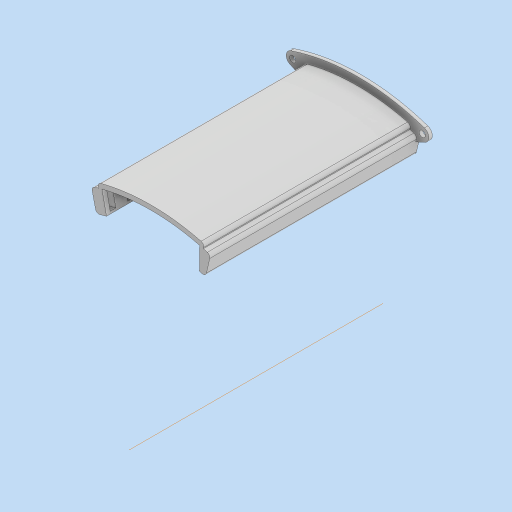
# Autodesk Inventor part: Shim_Tray
Saved by Autodesk Inventor 2024.2 (Build 282272000, 272)
## iProperties
Created: 2025-04-23
Part Number: Shim_Tray
Material: Generic
Document SubType Name: Modeling
Designer: 23661194
Density: 1 g/cm^3
Appearance: Default
Author: 23661194
Autodesk Inventor part; units mm, degrees
ref_plane "YZ Plane" through (0, 0, 0) normal (1, 0, 0) x (0, 1, 0)
ref_plane "XZ Plane" through (0, 0, 0) normal (0, 1, 0) x (-1, 0, 0)
sketch "Shim Tray Slot" plane through (0, 0, 0) normal (0, 0, 1) x (1, 0, 0)
  arc A0 (-28.6337, 111.3782) -> (-30.092, 109.0254) centre (-28.1357, 109.4412) ccw
  arc A1 (-31.6821, 97.1202) -> (-29.1504, 95.657) centre (-29.7334, 97.5701) ccw
  arc A2 (29.1504, 95.657) -> (31.6821, 97.1202) centre (29.7309, 97.5743) ccw
  arc A3 (33.5758, 105.3229) -> (32.2001, 107.689) centre (31.6271, 105.7728) ccw
  arc A4 (30.092, 109.0254) -> (28.6337, 111.3782) centre (28.1357, 109.4412) ccw
  line L0 (30.092, 109.0254) -> (29.9458, 108.3375)
  line L1 (33.5758, 105.3229) -> (31.6821, 97.1202)
  line L2 (-33.5758, 105.3229) -> (-31.6821, 97.1202)
  line L3 (-30.092, 109.0254) -> (-29.9458, 108.3375)
  arc A5 (-32.2001, 107.689) -> (-33.5758, 105.3229) centre (-31.6271, 105.7728) ccw
  arc A6 (29.1504, 95.657) -> (-29.1504, 95.657) centre (0, 0) ccw
  arc A7 (28.6337, 111.3782) -> (-28.6337, 111.3782) centre (0, 0) ccw
  arc A8 (-29.9458, 108.3375) -> (-32.2001, 107.689) centre (0, 0) ccw
  arc A9 (32.2001, 107.689) -> (29.9458, 108.3375) centre (0, 0) ccw
  line L4 (0, 0) -> (0, 107.5)
sketch "Sketch1" plane through (0, 0, 0) normal (0, 0, 1) x (1, 0, 0)
  circle A0 centre (0, 0) radius 100
  circle A1 centre (0, 0) radius 115
  line L0 (0, 161) -> (0, -161) projected
  line L1 (-34.5812, 109.6774) -> (-31.1949, 95.0099)
  line L2 (-161, 0) -> (161, 0) projected
  line L3 (34.5812, 109.6774) -> (31.1949, 95.0099)
  circle A2 centre (0, 0) radius 112.4
  line L4 (-25.4301, 96.7125) -> (-28.0109, 108.8538)
  line L5 (-29.9458, 108.3375) -> (-30.4873, 110.8852)
  arc A3 (-29.9458, 108.3375) -> (-33.9944, 107.1361) centre (0, 0) ccw
  arc A4 (-25.4301, 96.7125) -> (-31.1949, 95.0099) centre (0, 0) ccw
  line L6 (25.4301, 96.7125) -> (28.0109, 108.8538)
  line L7 (29.9458, 108.3375) -> (30.4873, 110.8852)
  arc A5 (31.1949, 95.0099) -> (25.4301, 96.7125) centre (0, 0) ccw
  arc A6 (33.9944, 107.1361) -> (29.9458, 108.3375) centre (0, 0) ccw
  arc A7 (28.0109, 108.8538) -> (-28.0109, 108.8538) centre (0, 0) ccw
  arc A8 (30.4873, 110.8852) -> (-30.4873, 110.8852) centre (0, 0) ccw
  circle A9 centre (0, 0) radius 101.2
  circle A10 centre (0, 0) radius 110.8
  line L8 (28.0109, 108.8538) -> (27.6779, 107.2873)
  line L9 (27.6779, 107.2873) -> (27.7719, 97.3148)
  line L10 (27.7719, 97.3148) -> (27.5218, 96.1382)
  circle A11 centre (0, 0) radius 107.5
  point P0 (0, 107.5)
  dimension "d41" = 202.4
  dimension "d42" = 221.6
  dimension "d53" = 215
  dimension "d0" = 200
  dimension "d1" = 230
  dimension "d4" = 69.1623
  dimension "d5" = 34.5812
  dimension "d6" = 34.5812
  dimension "d7" = 77
  dimension "d8" = 77
  dimension "d9" = 224.8
  dimension "d10" = 6
  dimension "d11" = 78
  dimension "d13" = 2
  dimension "d14" = 6
  dimension "d15" = 78
  dimension "d17" = 2
  dimension "d43" = 0.54
  dimension "d44" = -12
  constraints: 25 point on circle, 18 coincident, 18 end point, 9 centre point, 4 point on line, 1 midpoint, 1 vertical alignment, 8 other
  measures "d0" diameter of A0
  measures "d1" diameter of A1
  measures "d4" distance of L3.start L1.start
  measures "d5" distance from line of L0 L1.start
  measures "d6" distance from line of L0 L3.start
  measures "d7" angle of L2 L1
  measures "d8" angle of L2 L3
  measures "d9" diameter of A2
  measures "d10" distance from line of L4.start L1
  measures "d11" angle of L2 L4
  measures "d13" distance between parallel lines of L4 L5
  measures "d14" distance from line of L6.start L3
  measures "d15" angle of L2 L6
  measures "d17" distance between parallel lines of L6 L7
  measures "d43" angle of L0 L9
  measures "d44" angle of L0 L10
extrude "Extrusion1" add sketch "Sketch1" along normal blind 118 contours A0 L10 A9 L3 | A9 L9 A11 L3 | A11 L9 A10 L3 | L1 A9 L4 A0 | A10 L6 A2 L3 | L1 A11 L4 A9 | L1 A10 L4 A11 | A2 L0 A1 L7 | L1 A2 L4 A10 | A2 L5 A1 L0
fillet "Fillet1" radius 2 6 edges at (-33.9944, 107.1361, 59) (-31.1949, 95.0099, 59) (-30.4873, 110.8852, 59) (30.4873, 110.8852, 59) (33.9944, 107.1361, 59) (31.1949, 95.0099, 59)
ref_plane "Work Plane2" through (0, 0, 5.6) normal (0, 0, 1) x (1, 0, 0)
sketch "Sketch3" plane through (0, 0, 5.6) normal (0, 0, 1) x (1, 0, 0)
  circle A0 centre (0, 0) radius 101.2
  circle A1 centre (0, 0) radius 110.8
  line L0 (-25.4301, 96.7125) -> (-28.0109, 108.8538) projected
  line L1 (-25.6799, 97.8876) -> (-27.6779, 107.2873)
  line L2 (-33.5758, 105.3229) -> (-31.6821, 97.1202) projected
  line L3 (-29.7447, 96.73) -> (-31.9092, 106.1058)
  line L4 (31.6821, 97.1202) -> (33.5758, 105.3229) projected
  line L5 (29.7447, 96.73) -> (31.9092, 106.1058)
  line L6 (27.6779, 107.2873) -> (25.6799, 97.8876)
  line L7 (0, 160.16) -> (0, -155.96) projected
  arc A2 (31.9092, 106.1058) -> (27.6779, 107.2873) centre (0, 0) ccw
  arc A3 (29.7447, 96.73) -> (25.6799, 97.8876) centre (0, 0) ccw
  dimension "d30" = 202.4
  dimension "d31" = 221.6
  dimension "d32" = 1.8
  dimension "d33" = 1.8
  dimension "d45" = 1.8
  dimension "d46" = 1.8
  dimension "d47" = 12
  constraints: 12 point on circle, 8 end point, 4 centre point, 4 coincident, 2 point on line
  measures "d30" diameter of A0
  measures "d31" diameter of A1
  measures "d32" distance from line of L2 L3.start
  measures "d33" distance from line of L2 L3.end
  measures "d45" distance from line of L4 L5.end
  measures "d46" distance from line of L4 L5.start
  measures "d47" angle of L7 L6
extrude "Extrusion3" cut sketch "Sketch3" against normal blind 3.2 contours A0 L6 A1 L5 | L3 A1 L0 A0
fillet "Fillet2" radius 1 2 edges at (-31.9092, 106.1058, 4) (31.9092, 106.1058, 4)
pattern_linear "Rectangular Pattern1" count 12 spacing 10 along (0, 0, 1) of "Extrusion3", "Fillet2"
sketch "Sketch5" plane through (0, 0, 118) normal (0, 0, 1) x (1, 0, 0)
  arc A0 (-25.4301, 96.7125) -> (-29.1504, 95.657) centre (0, 0) ccw projected
  arc A1 (-28.6337, 111.3782) -> (-30.092, 109.0254) centre (-28.1357, 109.4412) ccw projected
  arc A2 (-31.6821, 97.1202) -> (-29.1504, 95.657) centre (-29.7334, 97.5701) ccw projected
  arc A3 (33.5758, 105.3229) -> (32.2001, 107.689) centre (31.6271, 105.7728) ccw projected
  arc A4 (30.092, 109.0254) -> (28.6337, 111.3782) centre (28.1357, 109.4412) ccw projected
  line L0 (29.9458, 108.3375) -> (30.092, 109.0254) projected
  line L1 (-33.5758, 105.3229) -> (-31.6821, 97.1202) projected
  line L2 (-30.092, 109.0254) -> (-29.9458, 108.3375) projected
  arc A5 (-32.2001, 107.689) -> (-33.5758, 105.3229) centre (-31.6271, 105.7728) ccw projected
  line L3 (-25.4301, 96.7125) -> (-28.0109, 108.8538) projected
  arc A6 (28.0109, 108.8538) -> (-28.0109, 108.8538) centre (0, 0) ccw
  arc A7 (-29.9458, 108.3375) -> (-32.2001, 107.689) centre (0, 0) ccw projected
  circle A8 centre (0, 0) radius 107.5
  arc A9 (-28.6337, 111.3782) -> (-30.092, 109.0254) centre (-28.1357, 109.4412) ccw
  arc A10 (-31.6821, 97.1202) -> (-29.1504, 95.657) centre (-29.7334, 97.5701) ccw
  arc A11 (29.1504, 95.657) -> (31.6821, 97.1202) centre (29.7309, 97.5743) ccw
  arc A12 (33.5758, 105.3229) -> (32.2001, 107.689) centre (31.6271, 105.7728) ccw
  arc A13 (30.092, 109.0254) -> (28.6337, 111.3782) centre (28.1357, 109.4412) ccw
  line L4 (30.092, 109.0254) -> (29.9458, 108.3375)
  line L5 (33.5758, 105.3229) -> (31.6821, 97.1202)
  line L6 (-33.5758, 105.3229) -> (-31.6821, 97.1202)
  line L7 (-30.092, 109.0254) -> (-29.9458, 108.3375)
  arc A14 (-32.2001, 107.689) -> (-33.5758, 105.3229) centre (-31.6271, 105.7728) ccw
  arc A15 (29.1504, 95.657) -> (-29.1504, 95.657) centre (0, 0) ccw
  arc A16 (28.6337, 111.3782) -> (-28.6337, 111.3782) centre (0, 0) ccw
  arc A17 (-29.9458, 108.3375) -> (-32.2001, 107.689) centre (0, 0) ccw
  arc A18 (32.2001, 107.689) -> (29.9458, 108.3375) centre (0, 0) ccw
  line L8 (0, 0) -> (0, 107.5)
  dimension "d55" = 215
  constraints: 2 centre point, 2 point on circle, 8 other
  measures "d55" diameter of A8
sketch "Sketch6" plane through (0, 0, 0) normal (0, 0, 1) x (1, 0, 0)
  arc A0 (29.1504, 95.657) -> (27.5218, 96.1382) centre (0, 0) ccw projected
  arc A1 (29.1504, 95.657) -> (-29.1504, 95.657) centre (0, 0) ccw
  arc A2 (28.6337, 111.3782) -> (-28.6337, 111.3782) centre (0, 0) ccw projected
  arc A3 (28.6337, 111.3782) -> (-28.6337, 111.3782) centre (0, 0) ccw
  arc A4 (30.092, 109.0254) -> (28.6337, 111.3782) centre (28.1357, 109.4412) ccw projected
  arc A5 (30.092, 109.0254) -> (28.6337, 111.3782) centre (28.1357, 109.4412) ccw
  arc A6 (33.5758, 105.3229) -> (32.2001, 107.689) centre (31.6271, 105.7728) ccw projected
  arc A7 (33.5758, 105.3229) -> (32.2001, 107.689) centre (31.6271, 105.7728) ccw
  arc A8 (29.1504, 95.657) -> (31.6821, 97.1202) centre (29.7334, 97.5701) ccw projected
  arc A9 (29.1504, 95.657) -> (31.6821, 97.1202) centre (29.7334, 97.5701) ccw
  arc A10 (-31.6821, 97.1202) -> (-29.1504, 95.657) centre (-29.7334, 97.5701) ccw projected
  arc A11 (-31.6821, 97.1202) -> (-29.1504, 95.657) centre (-29.7334, 97.5701) ccw
  arc A12 (-28.6337, 111.3782) -> (-30.092, 109.0254) centre (-28.1357, 109.4412) ccw projected
  arc A13 (-28.6337, 111.3782) -> (-30.092, 109.0254) centre (-28.1357, 109.4412) ccw
  arc A14 (-32.2001, 107.689) -> (-33.5758, 105.3229) centre (-31.6271, 105.7728) ccw projected
  arc A15 (-32.2001, 107.689) -> (-33.5758, 105.3229) centre (-31.6271, 105.7728) ccw
  arc A16 (32.2001, 107.689) -> (29.9458, 108.3375) centre (0, 0) ccw projected
  line L0 (32.2001, 107.689) -> (29.9458, 108.3375)
  line L1 (29.9458, 108.3375) -> (30.092, 109.0254)
  line L2 (33.5758, 105.3229) -> (31.6821, 97.1202)
  line L3 (-33.5758, 105.3229) -> (-31.6821, 97.1202) projected
  line L4 (-31.6821, 97.1202) -> (-33.5758, 105.3229)
  line L5 (-30.092, 109.0254) -> (-29.9458, 108.3375) projected
  line L6 (-30.092, 109.0254) -> (-29.9458, 108.3375)
  arc A17 (-29.9458, 108.3375) -> (-32.2001, 107.689) centre (0, 0) ccw projected
  line L7 (-29.9458, 108.3375) -> (-32.2001, 107.689)
  arc A18 (47.2152, 105.6825) -> (0, 115.75) centre (0, 0) ccw
  circle A19 centre (37, 109.6771) radius 1.75
  arc A20 (0, 115.75) -> (-45.3069, 106.5145) centre (0, 0) ccw
  circle A21 centre (-37, 109.6771) radius 1.75
  line L8 (0, 163.6931) -> (0, -152.6989) projected
  circle A22 centre (37, 109.6771) radius 3.75
  circle A23 centre (-37, 109.6771) radius 3.75
  line L9 (0, 0) -> (37, 109.6771)
  line L10 (37, 109.6771) -> (38.1987, 113.2303)
  line L11 (0, 0) -> (-37, 109.6771)
  arc A24 (38.1987, 113.2303) -> (-38.1987, 113.2303) centre (0, 0) ccw
  circle A25 centre (0, 0) radius 109
  line L12 (33.2271, 103.8122) -> (38, 106.0629)
  line L13 (-33.2271, 103.8122) -> (-38, 106.0629)
  point P0 (-33.2271, 103.8122)
  point P1 (27.5218, 96.1382)
  dimension "d56" = 115.75
  dimension "d57" = 3.5
  dimension "d58" = 3.5
  dimension "d59" = 37
  dimension "d60" = 37
  dimension "d61" = 7.5
  dimension "d62" = 7.5
  dimension "d63" = 218
  constraints: 31 point on circle, 22 end point, 16 centre point, 13 coincident, 2 collinear, 2 point on line
  measures "d56" radius of A18
  measures "d57" diameter of A19
  measures "d58" diameter of A21
  measures "d59" distance from line of L8 A19.centre
  measures "d60" distance from line of L8 A21.centre
  measures "d61" diameter of A22
  measures "d62" diameter of A23
  measures "d63" diameter of A25
extrude "Extrusion4" add sketch "Sketch6" against normal blind 2 contours A0 A1 L8 A25 L2 A8 | A1 A10 L3 A25 L8 | A25 L8 A2 A4 L1 L0 A6 L2 | L2 A6 A16 L1 A4 A2 L8 A18 A22 L9 L12 | A25 L3 A14 L7 L5 A12 A2 L8 | L9 A22 L12 | A2 A12 L5 A17 A14 L3 L13 L11 A23 A20 L8 | L0 A16 | L9 A19 A18 A22 | A22 A18 A19 L9 | L8 A24 A22 A18 | A20 A23 A24 L8 | L13 A23 L11 | A22 L10 A19 A18 | A18 A19 L10 A22 | A23 L11 A21 A20 | A20 A21 A23 | A17 L7 | A23 A20 A21 L11
sketch "Sketch7" plane through (0, 0, 0) normal (0, 0, 1) x (1, 0, 0)
  arc A0 (27.5218, 96.1382) -> (-25.4301, 96.7125) centre (0, 0) ccw projected
  line L0 (0, 164.9) -> (0, -152.9) projected
  line L1 (0, 100) -> (-6.0909, 111.9541)
  line L2 (0, 100) -> (6.0909, 111.9541)
  arc A1 (6.0909, 111.9541) -> (-6.0909, 111.9541) centre (0, 0) ccw
  point P0 (0, 100)
  dimension "d67" = 27
  dimension "d69" = 27
  constraints: 4 end point, 3 point on circle, 2 point on line, 1 centre point, 1 coincident
  measures "d67" angle of L0 L1
  measures "d69" angle of L0 L2
extrude "Extrusion5" cut sketch "Sketch7" against normal blind 2
thicken "Thicken1" operation cut thickness 0.5 both sides no extend neighbours no toward (0.8910065, -0.4539905, 0) faces at (2.0303, 103.9847, -0.6667) (-4.0606, 107.9694, -0.6667)
fillet "Fillet3" radius 1 6 edges at (0.5604, 99.9984, -1) (-0.5604, 99.9984, -1) (6.0909, 111.9541, -1) (6.5364, 111.7271, -1) (-6.0909, 111.9541, -1) (-6.5364, 111.7271, -1)
body "Solid1"
